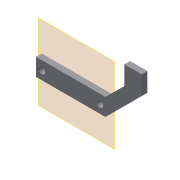
# Autodesk Inventor part: 10_MiniSPIM_Sampleholder
Saved by Autodesk Inventor 2019 (Build 230136000, 136)
## iProperties
Created: 2019-10-13
Part Number: 10_MiniSPIM_Sampleholder
Material: Generic
Document SubType Name: Modeling
Designer: diederichbenedict
Density: 1 g/cm^3
Appearance: Default
Author: diederichbenedict
Autodesk Inventor part; units mm, degrees
ref_plane "YZ Plane" through (0, 0, 0) normal (1, 0, 0) x (0, 1, 0)
ref_plane "XZ Plane" through (0, 0, 0) normal (0, 1, 0) x (-1, 0, 0)
ref_plane "XY Plane" through (0, 0, 0) normal (0, 0, 1) x (1, 0, 0)
ref_plane "Work Plane1" through (0, 0, 0) normal (0, 0, 1) x (1, 0, 0)
sketch "Sketch1" plane through (0, 0, 0) normal (0, 0, 1) x (1, 0, 0)
  line L0 (28, 30) -> (30, 28) construction
  line L1 (28, 30) -> (-28, 30) construction
  line L2 (-30, 28) -> (-28, 30) construction
  line L3 (-30, 28) -> (-30, -28) construction
  line L4 (-28, -30) -> (-30, -28) construction
  line L5 (-28, -30) -> (28, -30) construction
  line L6 (30, -28) -> (28, -30) construction
  line L7 (30, -28) -> (30, 28) construction
  circle A0 centre (25, 0) radius 1.3 construction
  circle A1 centre (-25, 0) radius 1.3 construction
  circle A2 centre (0, 0) radius 7.5 construction
  line L8 (-30, -7.5) -> (40, -7.5)
  line L9 (40, -7.5) -> (40, 7.5)
  line L10 (40, 7.5) -> (-30, 7.5)
  line L11 (-30, 7.5) -> (-30, -7.5)
  line L12 (40, -7.5) -> (66.2425, 18.7425)
  line L13 (40, -7.5) -> (77.1125, -7.5) construction
  line L14 (66.2425, 18.7425) -> (66.2425, 27.2511)
  line L15 (40, 7.5) -> (56.2425, 23.7425)
  line L16 (40, 7.5) -> (62.9703, 7.5) construction
  line L17 (56.2425, 23.7425) -> (56.2425, 27.2511)
  line L18 (66.2425, 27.2511) -> (66.2425, 33.815)
  line L19 (66.2425, 33.815) -> (56.2425, 33.815)
  line L20 (56.2425, 33.815) -> (56.2425, 27.2511)
  circle A3 centre (-25, 0) radius 2
  circle A4 centre (25, 0) radius 2
  circle A5 centre (61.2425, 28.815) radius 3.5
  line L21 (79.415, 27.3813) -> (49.415, 27.3813) construction
  line L22 (79.415, 30.2423) -> (49.415, 30.2423) construction
  line L23 (62.6454, 27.3813) -> (62.6454, -21.1882) construction
  line L24 (59.7845, 27.3813) -> (59.7845, -21.1882) construction
  point P0 (0, 0)
  dimension "d0" = 70
  dimension "d1" = 45
  dimension "d2" = 45
  dimension "d3" = 10
  dimension "d4" = 15
  dimension "d5" = 7.5
  dimension "d7" = 4
  dimension "d8" = 4
  dimension "d11" = 7
  dimension "d12" = 5
  dimension "d13" = 5
  constraints: 34 end point, 5 horizontal, 4 vertical, 3 centre point, 3 parallel, 2 coincident, 2 equal length, 1 perpendicular, 1 point on line, 8 other
  measures "d0" distance of L10.end L9.end
  measures "d1" angle of L13 L12
  measures "d2" angle of L16 L15
  measures "d3" distance between parallel lines of L14 L17
  measures "d4" distance between parallel lines of L8 L10
  measures "d5" distance from line of point (0, 0) L10
  measures "d7" diameter of A3
  measures "d8" diameter of A4
  measures "d11" diameter of A5
  measures "d12" distance from line of A5.centre L14
  measures "d13" distance from line of A5.centre L19
extrude "Extrusion1" add sketch "Sketch1" along normal blind 5
fillet "Fillet1" radius 4 6 edges at (40, 7.5, 2.5) (56.2425, 33.815, 2.5) (66.2425, 33.815, 2.5) (66.2425, 18.7425, 2.5) (40, -7.5, 2.5) (56.2425, 23.7425, 2.5)
body "Solid1"
